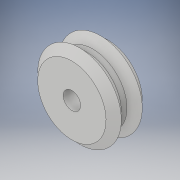
# Autodesk Inventor part: bearingType2Standin
Saved by Autodesk Inventor 2019 (Build 230136000, 136)
## iProperties
Created: 2019-05-08
Part Number: bearingType2Standin
Material: Generic
Document SubType Name: Modeling
Designer: Alex Jones
Density: 1 g/cm^3
Appearance: Default
Author: Alex Jones
Autodesk Inventor part; units mm, degrees
ref_plane "YZ Plane" through (0, 0, 0) normal (1, 0, 0) x (0, 1, 0)
ref_plane "XZ Plane" through (0, 0, 0) normal (0, 1, 0) x (-1, 0, 0)
ref_plane "XY Plane" through (0, 0, 0) normal (0, 0, 1) x (1, 0, 0)
sketch "Sketch1" plane through (0, 0, 0) normal (1, 0, 0) x (0, 1, 0)
  line L0 (0, 0) -> (0, -15.044)
  line L1 (2.5, 0) -> (2.5, -12.9861)
  line L2 (0, -7.522) -> (12, -7.522) construction
  line L3 (0, -1.512) -> (12, -1.512) construction
  line L4 (12, -1.512) -> (9.805, 0.683)
  line L5 (12, -7.522) -> (9.805, -9.717)
  line L6 (12, -1.512) -> (9.805, -3.707)
  line L7 (12, -7.522) -> (9.805, -5.327)
  line L8 (9.805, -5.327) -> (9.805, -3.707)
  line L9 (9.805, 0.683) -> (2.5, 0.683)
  line L10 (2.5, 0.683) -> (2.5, 0)
  line L11 (9.805, -9.717) -> (2.5, -9.717)
  dimension "d0" = 2.5
  dimension "d1" = 12
  dimension "d2" = 6.01
  dimension "d3" = 45
  dimension "d4" = 0
  dimension "d5" = 10.4
  constraints: 24 end point, 4 perpendicular, 3 horizontal, 2 point on line, 2 vertical, 1 midpoint, 1 parallel
  measures "d0" distance between parallel lines of L0 L1
  measures "d1" distance of L2.start L2.end
  measures "d2" distance between parallel lines of L2 L3
  measures "d3" angle of L2 L5
  measures "d4" horizontal distance of L2.end L3.end
  measures "d5" distance of L5.end L4.end
revolve "Revolution1" add sketch "Sketch1" angle 360 about axis through (0, 0, 0) along (0, 0, -1)
body "Solid1"
